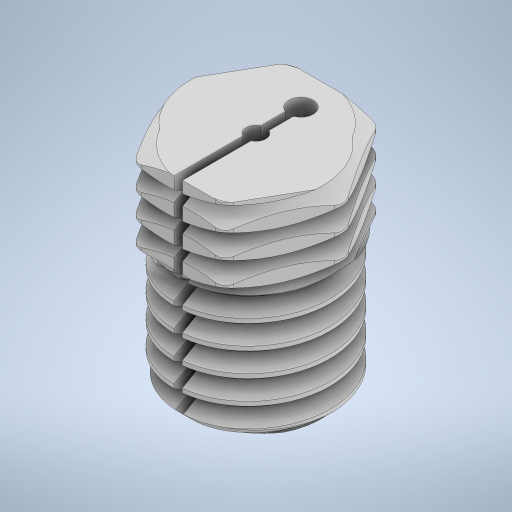
# Autodesk Inventor part: Proyectos trabajo UNIANDES
Saved by Autodesk Inventor 2024.2 (Build 282272000, 272)
## iProperties
Created: 2025-08-07
Part Number: Proyectos trabajo UNIANDES
Material: Genérico
Document SubType Name: Modeling
Designer: ja.restrepo1
Density: 1 g/cm^3
Appearance: Valor por defecto
Author: ja.restrepo1
Autodesk Inventor part; units mm, degrees
ref_plane "YZ Plane" through (0, 0, 0) normal (1, 0, 0) x (0, 1, 0)
ref_plane "XY Plane" through (0, 0, 0) normal (0, 0, 1) x (1, 0, 0)
sketch "Boceto1" plane through (0, 0, 0) normal (1, 0, 0) x (0, 1, 0)
  line L0 (4.9, 5.7) -> (-4.9, 5.7)
  line L1 (-4.9, 5.7) -> (-4.9, 0.725)
  line L2 (-4.9, 0.725) -> (4.9, 0.725)
  line L3 (4.9, 0.725) -> (4.9, 5.7)
  line L4 (-6.86, 0) -> (6.86, 0) projected
  point P0 (0, 0)
  point P1 (0, 0.725)
  dimension "d3" = 0.725
  dimension "d4" = 9.8
  dimension "d5" = 5.7
  constraints: 8 end point, 2 parallel, 1 horizontal, 1 midpoint, 1 perpendicular, 1 vertical alignment
  measures "d3" distance from line of point (0, 0) L2
  measures "d4" distance of L0.start L0.end
  measures "d5" distance from line of point (0, 0) L0
revolve "cuerpo ferula O" add sketch "Boceto1" angle 360 about axis through (0, -10, 0) along (0, 1, 0)
chamfer "60°" distance 1 angle 45 1 edges at (0, -4.9, -5.7)
sketch "Boceto2" plane through (0, 0, 0) normal (0, 0, 1) x (1, 0, 0)
  line L0 (0, -9) -> (-4.45, -9) construction
  line L1 (-4.6, -9.0866) -> (-5.8695, -9.8195)
  line L2 (-5.8695, -9.8195) -> (-5.8695, -8.1804)
  line L3 (-5.8695, -8.1804) -> (-4.6, -8.9134)
  arc A0 (-4.6, -9.0866) -> (-4.6, -8.9134) centre (-4.65, -9) ccw
  point P0 (0, 0)
  point P1 (-5.3963, -9)
  dimension "d10" = 4.45
  dimension "d11" = 9
  dimension "d12" = 1.6391
  dimension "d13" = 0.1
  constraints: 8 end point, 2 point on circle, 2 point on line, 2 tangent, 1 centre point, 1 horizontal, 1 vertical, 1 vertical alignment, 7 other
  measures "d10" distance of L0.start L0.end
  measures "d11" distance from line of point (0, 0) L0
  measures "d12" distance of L1.end L2.end
  measures "d13" radius of A0
coil "M12" sketch "Boceto2" operation cut axis through (0, -10, 0) along (0, 1, 0) pitch 1.75 turns 10 hand right
ref_plane "Plano de trabajo1" through (0, 6.9, 0) normal (0, 1, 0) x (-1, 0, 0)
sketch "Boceto3" plane through (0, 4.9, 0) normal (0, 1, 0) x (-1, 0, 0)
  circle A0 centre (0, 0) radius 0.725 projected
  line L0 (2.6991, -5.675) -> (-2.6991, -5.675)
  line L1 (-3.5651, -5.175) -> (-6.2643, -0.5)
  line L2 (-6.2643, 0.5) -> (-3.5651, 5.175)
  line L3 (-2.6991, 5.675) -> (2.6991, 5.675)
  line L4 (3.5651, 5.175) -> (6.2643, 0.5)
  line L5 (6.2643, -0.5) -> (3.5651, -5.175)
  arc A1 (6.2643, -0.5) -> (6.2643, 0.5) centre (5.3982, 0) ccw
  arc A2 (2.6991, -5.675) -> (3.5651, -5.175) centre (2.6991, -4.675) ccw
  arc A3 (-3.5651, -5.175) -> (-2.6991, -5.675) centre (-2.6991, -4.675) ccw
  arc A4 (-6.2643, 0.5) -> (-6.2643, -0.5) centre (-5.3982, 0) ccw
  arc A5 (-2.6991, 5.675) -> (-3.5651, 5.175) centre (-2.6991, 4.675) ccw
  arc A6 (3.5651, 5.175) -> (2.6991, 5.675) centre (2.6991, 4.675) ccw
  point P0 (3.2765, -5.675)
  point P1 (-3.2765, -5.675)
  point P2 (-6.5529, 0)
  point P3 (-3.2765, 5.675)
  point P4 (3.2765, 5.675)
  point P5 (6.5529, 0)
  dimension "d23" = 11.35
  dimension "d63" = 1
  constraints: 12 end point, 12 point on circle, 12 point on line, 12 tangent, 6 centre point, 5 equal radius, 1 coincident, 1 horizontal, 13 other
  measures "d23" distance between parallel lines of L0 L3
  measures "d63" radius of A1
extrude "Hexa 12" add sketch "Boceto3" along normal blind 6
sketch "Boceto4" plane through (0, 0, 0) normal (1, 0, 0) x (0, 1, 0)
  arc A0 (3.0412, -5.3877) -> (4.9, -5.9) centre (3.9, -5.9) ccw construction
  line L0 (-4.9, -4.7) -> (-4.9, -0.725) projected
  line L1 (-4.9, -0.725) -> (10.9, -0.725) projected
  line L2 (10.9, -0.725) -> (10.9, -5.675) projected
  line L3 (10.9, -5.675) -> (4.9, -5.675) projected
  line L4 (4.9, -5.675) -> (4.9, -5.0346) projected
  line L5 (-4.9, 0.725) -> (-4.9, 4.7) projected
  line L6 (4.9, 5.381) -> (4.9, 5.675) projected
  line L7 (4.9, 5.675) -> (10.9, 5.675) projected
  line L8 (10.9, 5.675) -> (10.9, 0.725) projected
  line L9 (10.9, 0.725) -> (-4.9, 0.725) projected
  arc A1 (4.1, -4.9202) -> (3.0412, -5.3877) centre (3.9, -5.9) ccw construction
  arc A2 (4.9, -5.9) -> (4.1, -4.9202) centre (3.9, -5.9) ccw
  line L10 (4.1, -4.9202) -> (4.1, -4.8)
  line L11 (4.1, -4.8) -> (4.9, -4.8)
  line L12 (4.9, -4.8) -> (4.9, -5.9)
  line L13 (-8.06, 0) -> (14.06, 0) projected
  line L14 (-2.5908, 5.7) -> (-2.2842, 5.7) projected
  line L15 (-0.8408, 5.7) -> (-0.5342, 5.7) projected
  line L16 (0.9092, 5.7) -> (1.2158, 5.7) projected
  line L17 (2.6592, 5.7) -> (2.9658, 5.7) projected
  line L18 (4.4092, 5.7) -> (4.7158, 5.7) projected
  line L19 (-4.9, 4.7) -> (-3.9851, 5.6149) projected
  line L20 (-4.5398, -5.0602) -> (-4.9, -4.7) projected
  line L21 (3.8408, -5.7) -> (3.5342, -5.7) projected
  line L22 (2.0908, -5.7) -> (1.7842, -5.7) projected
  line L23 (0.3408, -5.7) -> (0.0342, -5.7) projected
  line L24 (-1.4092, -5.7) -> (-1.7158, -5.7) projected
  line L25 (-3.1592, -5.7) -> (-3.4658, -5.7) projected
  point P0 (0, 0)
  point P1 (4.9, -5.1346)
  point P2 (4.9, -5.1346)
  point P3 (4.9, 5.481)
  point P4 (4.2633, -4.9683)
  point P5 (4.3604, -4.8)
  point P6 (4.4759, -4.7)
  point P7 (4.6491, -4.7)
  point P8 (4.7646, -4.8)
  point P9 (4.9, -5.1346)
  dimension "d30" = 2
  dimension "d32" = 1.1
  dimension "d64" = 4.8
  dimension "d65" = 0.8
  constraints: 10 horizontal alignment, 6 end point, 6 point on circle, 3 centre point, 3 tangent, 2 perpendicular, 1 point on line, 1 vertical, 24 other
  measures "d30" diameter of A0
  measures "d32" distance from line of L11 L12.end
  measures "d64" distance from line of point (0, 0) L11
  measures "d65" distance of L10.end L11.end
revolve "empalme rosca hexa" add sketch "Boceto4" angle 360 about axis through (0, -10, 0) along (0, 1, 0)
sketch "Boceto5" plane through (0, 10.9, 0) normal (0, 1, 0) x (1, 0, 0)
  arc A0 (0.3, 2.4515) -> (-0.3, 2.4515) centre (0, 3.3) ccw
  line L0 (-0.3, 3.3) -> (0.3, 3.3) construction
  line L1 (0.3, 3.3) -> (0.3, 2.4515) construction
  line L2 (0.3, -6.1485) -> (-0.3, -6.1485)
  line L3 (-0.3, -6.1485) -> (-0.3, 2.4515)
  line L4 (-0.3, 2.4515) -> (-0.3, 3.3) construction
  line L5 (0.3, 2.4515) -> (0.3, -6.1485)
  arc A1 (-0.3, 2.4515) -> (0.3, 2.4515) centre (0, 3.3) ccw construction
  point P0 (0, 0)
  dimension "d34" = 1.8
  dimension "d35" = 0.6
  dimension "d36" = 3.3
  dimension "d37" = 8.6
  constraints: 12 end point, 5 parallel, 4 point on circle, 2 centre point, 2 coincident, 2 perpendicular, 1 horizontal, 1 midpoint, 1 vertical alignment
  measures "d34" diameter of A0
  measures "d35" distance of L2.start L2.end
  measures "d36" distance of A0.centre point (0, 0)
  measures "d37" distance of L1.end L2.start
extrude "Extrusión2" cut sketch "Boceto5" against normal through all
sketch "Boceto6" plane through (0, 0, 0) normal (0, 0, 1) x (1, 0, 0)
  line L0 (0, 14) -> (-5, 14) construction
  line L1 (-5, 14) -> (-6.4266, 13.1764)
  line L2 (-6.4266, 13.1764) -> (-6.4266, 14.8237)
  line L3 (-6.4266, 14.8237) -> (-5, 14)
  line L4 (0, 14) -> (5, 14) construction
  line L5 (6.4266, 14.8237) -> (6.4266, 13.1764)
  line L6 (6.4266, 13.1764) -> (5, 14)
  line L7 (5, 14) -> (6.4266, 14.8237)
  point P0 (0, 0)
  point P1 (-5.9511, 14)
  point P2 (5.9511, 14)
  dimension "d40" = 5
  dimension "d41" = 14
  dimension "d42" = 1.6473
  dimension "d44" = 5
  dimension "d46" = 1.6473
  constraints: 16 end point, 2 horizontal, 2 vertical, 2 vertical alignment, 1 collinear, 14 other
  measures "d40" distance of L0.start L0.end
  measures "d41" distance from line of point (0, 0) L0
  measures "d42" distance of L1.end L2.end
  measures "d44" distance of L4.start L4.end
  measures "d46" distance of L5.start L5.end
coil "M12 2 IN" sketch "Boceto6" operation cut axis through (0, -10, 0) along (0, -1, 0) pitch 3.5 turns 2.8 hand right contours L1 L2 L3
coil "M12 2 IN F" sketch "Boceto6" operation cut axis through (0, -10, 0) along (0, -1, 0) pitch 3.5 turns 2.8 hand right contours L5 L6 L7
sketch "Sketch7" plane through (0, 0, 0) normal (0, 0, 1) x (1, 0, 0)
  line L0 (0, 7) -> (0, -8)
  line L1 (-0.3, 10.9) -> (-0.3, -4.9) projected
  line L2 (0, -8) -> (-3.8, -8)
  line L3 (-3.8, -8) -> (-2.2234, 7)
  line L4 (-2.2234, 7) -> (0, 7)
  point P0 (0, 0)
  point P1 (0, -0.5)
  dimension "d66" = 15
  dimension "d67" = 84
  dimension "d68" = 8
  dimension "d69" = 3.8
  constraints: 8 end point, 2 parallel, 1 midpoint, 1 perpendicular, 1 vertical alignment
  measures "d66" distance of L0.start L0.end
  measures "d67" angle of L2 L3
  measures "d68" distance from line of L2 point (0, 0)
  measures "d69" distance of L0.end L2.end
revolve "Revolution3" cut sketch "Sketch7" angle 360 about axis through (0, 7, 0) along (0, -1, 0)
equation "\"d44\" = d40"
equation "\"d46\" = d42"
